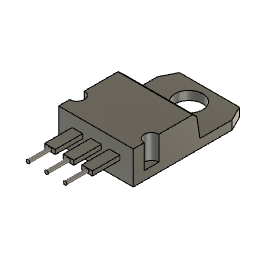
TO-220_Dgauge_Vertical (Autodesk Fusion 360 design; units mm, degrees)
Autodesk Fusion 360 part; units mm, degrees
sketch "スケッチ1" plane through (0, 0, 0) normal (0, 0, 1) x (1, 0, 0)
  line L0 (-5.1, -7.75) -> (5.1, -7.75)
  line L1 (5.1, -7.75) -> (5.1, 7.75)
  line L2 (5.1, 7.75) -> (-5.1, 7.75)
  line L3 (-5.1, 7.75) -> (-5.1, -7.75)
  circle A0 centre (0, 4.95) radius 1.9
  line L4 (0, 10.099) -> (0, 5.401) construction
  line L5 (6.6, 0) -> (3.6, 0) construction
  line L6 (1.75, 0) -> (22.5, 0)
  line L7 (0, 1.75) -> (0, 22.5)
  dimension "d1" = 10.2
  dimension "d2" = 15.5
  dimension "d5" = 3.8
  dimension "d6" = 2.8
  constraint horizontal L0
  constraint vertical L1
  constraint horizontal L2
  constraint vertical L3
  constraint vertical L4
  constraint midpoint L2 L4
  constraint coincident A0.centre L4
  constraint perpendicular L1 L5
  constraint midpoint L1 L5
  constraint collinear L5 L6
  constraint collinear L4 L7
  measures "d1" distance of L0.start L0.end
  measures "d2" distance of L0.start L2.end
  measures "d5" diameter of A0
  measures "d6" distance of L2 A0.centre
extrude "押し出し1" add sketch "スケッチ1" along normal blind 1.2
sketch "スケッチ2" plane through (0, 0, 1.2) normal (0, 0, 1) x (-1, 0, 0)
  circle A0 centre (0, -4.95) radius 1.9
  line L0 (5.1, -7.75) -> (5.1, 7.75)
  line L1 (5.1, 7.75) -> (-5.1, 7.75)
  line L2 (-5.1, 7.75) -> (-5.1, -7.75)
  line L3 (-5.1, -7.75) -> (5.1, -7.75)
  line L4 (5.1, -1.35) -> (-5.1, -1.35)
  line L5 (-5.1, -1.35) -> (-5.1, 7.75)
  line L6 (-5.1, 7.75) -> (5.1, 7.75)
  line L7 (5.1, 7.75) -> (5.1, -1.35)
  dimension "d7" = 6.4
  constraint horizontal L4
  constraint vertical L5
  constraint horizontal L6
  constraint vertical L7
  constraint collinear L1 L6
  constraint equal L1 L6
  constraint collinear L0 L7
  measures "d7" distance of L3 L4
extrude "押し出し2" add sketch "スケッチ2" along normal blind 3.3 contours L0 L1 L2 L4 L5 L6 L7
chamfer "面取り1" distance 1 distance2 2 1 edges at (-5.1, 7.75, 0.6) measured on face at (-1.7, 7.75, 0.8)
chamfer "面取り2" distance 2 distance2 1 1 edges at (5.1, 7.75, 0.6) measured on face at (5.1, -4.7167, 1.9)
chamfer "面取り3" distance 0.5 distance2 3.3 1 edges at (0, 1.35, 4.5) measured on face at (-1.7, -1.6833, 4.5)
chamfer "面取り4" distance 0.5 angle 45 1 edges at (0, 0.85, 4.5)
sketch "スケッチ3" plane through (0, 0, 4.5) normal (0, 0, 1) x (-1, 0, 0)
  line L0 (-5.1, -0.35) -> (5.1, -0.35)
  line L1 (5.1, -0.35) -> (5.1, 7.75)
  line L2 (5.1, 7.75) -> (-5.1, 7.75)
  line L3 (-5.1, 7.75) -> (-5.1, -0.35)
  line L4 (1.5345, 5.25) -> (-2.4655, 5.25) construction
  arc A0 (5.1, 6.25) -> (5.1, 4.25) centre (5.1, 5.25) ccw
  arc A1 (-5.1, 4.25) -> (-5.1, 6.25) centre (-5.1, 5.25) ccw
  dimension "d17" = 2
  dimension "d18" = 2.5
  dimension "d19" = 2
  constraint coincident L1 A0.centre
  constraint coincident L3 A1.centre
  constraint perpendicular L1 L4
  constraint coincident A1.centre L4
  constraint coincident A0.centre L4
  constraint coincident L1 A0.end
  constraint coincident L1 A0.start
  constraint coincident L3 A1.end
  constraint coincident L3 A1.start
  measures "d17" diameter of A1
  measures "d18" distance of L2 L4
  measures "d19" diameter of A0
extrude "押し出し3" cut sketch "スケッチ3" against normal blind 3.3 contours L3 A1 | L1 A0
sketch "スケッチ4" plane through (0, -7.75, 0) normal (0, -1, 0) x (1, 0, 0)
  line L0 (-5.1, 0) -> (5.1, 0)
  line L1 (5.1, 0) -> (5.1, 4.5)
  line L2 (5.1, 4.5) -> (-5.1, 4.5)
  line L3 (-5.1, 4.5) -> (-5.1, 0)
  line L4 (-0.725, 2.86) -> (0.725, 2.86)
  line L5 (0.725, 2.86) -> (0.725, 2.26)
  line L6 (0.725, 2.26) -> (-0.725, 2.26)
  line L7 (-0.725, 2.26) -> (-0.725, 2.86)
  line L8 (-1.15, 2.56) -> (-0.3, 2.56) construction
  line L9 (0, 5.2056) -> (0, 3.7944) construction
  line L10 (0, 3.2405) -> (0, 2.4795) construction
  dimension "d22" = 1.45
  dimension "d23" = 0.6
  dimension "d24" = 2.56
  constraint horizontal L4
  constraint vertical L5
  constraint horizontal L6
  constraint vertical L7
  constraint horizontal L8
  constraint midpoint L7 L8
  constraint perpendicular L2 L9
  constraint midpoint L2 L9
  constraint vertical L10
  constraint midpoint L4 L10
  constraint collinear L9 L10
  measures "d22" distance of L4.start L4.end
  measures "d23" distance of L4.start L6.end
  measures "d24" distance of L0 L8
extrude "押し出し4" add sketch "スケッチ4" along normal blind 3.75 contours L4 L5 L6 L7
sketch "スケッチ6" plane through (0, -11.5, 0) normal (0, -1, 0) x (1, 0, 0)
  line L0 (-0.725, 2.26) -> (0.725, 2.26)
  line L1 (0.725, 2.26) -> (0.725, 2.86)
  line L2 (0.725, 2.86) -> (-0.725, 2.86)
  line L3 (-0.725, 2.86) -> (-0.725, 2.26)
  circle A0 centre (0, 2.56) radius 0.25
  line L4 (-0.975, 2.56) -> (-0.475, 2.56) construction
  line L5 (0, 2.9781) -> (0, 2.7419) construction
  dimension "d34" = 0.5
  constraint perpendicular L3 L4
  constraint perpendicular L2 L5
  constraint midpoint L3 L4
  constraint midpoint L2 L5
  constraint coincident A0.centre L5
  constraint coincident A0.centre L4
  measures "d34" diameter of A0
extrude "押し出し6" add sketch "スケッチ6" along normal blind 3 contours A0
pattern_linear "R パターン2" count 3 spacing 2.54 along (1, 0, 0) both ways of "押し出し4", "押し出し6"
